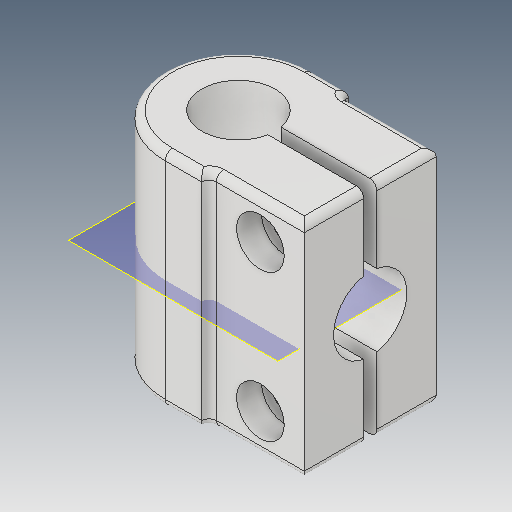
# Autodesk Inventor part: UpperArm_Yawn_Fixture
Saved by Autodesk Inventor 2021.4 (Build 254397000, 397)
## iProperties
Created: 2022-07-06
Part Number: UpperArm_Yawn_Fixture
Material: PBT Plastic
Document SubType Name: Modeling
Designer: alexw
Density: 1.31 g/cm^3
Appearance: Smooth - White
Mass: 13.7456 g
Surface Area: 52.7567 cm^2
Volume: 10.4928 cm^3
Author: alexw
Autodesk Inventor part; units mm, degrees
note: some values were not read from the file. Chosen so that the rebuilt part matches the saved one: direction of "Hole2".
ref_plane "YZ Plane" through (0, 0, 0) normal (1, 0, 0) x (0, 1, 0)
ref_plane "XZ Plane" through (0, 0, 0) normal (0, 1, 0) x (-1, 0, 0)
ref_plane "XY Plane" through (0, 0, 0) normal (0, 0, 1) x (1, 0, 0)
sketch "Sketch1" plane through (0, 0, 0) normal (0, 0, 1) x (1, 0, 0)
  line L0 (28, 30.2) -> (0, 30.2)
  line L1 (0, 30.2) -> (0, 0)
  line L2 (0, 15.1) -> (28, 15.1) construction
  line L3 (28, 0) -> (28, 30.2)
  line L4 (0, 0) -> (28, 0)
  line L5 (20, 15.1) -> (20, 30.2) construction
  dimension "d0" = 30.2
  dimension "d3" = 28
  dimension "d26" = 20
  dimension "d27" = 8
  constraints: 12 end point, 2 midpoint, 2 parallel, 2 perpendicular, 2 point on line, 1 horizontal, 1 symmetric about line
  measures "d0" distance of L0.end L1.end
  measures "d3" distance between parallel lines of L3 L1
  measures "d26" distance between parallel lines of L1 L5
  measures "d27" distance between parallel lines of L3 L5
extrude "Extrusion1" add sketch "Sketch1" along normal blind 20
sketch "Sketch2" plane through (0, 30.2, 0) normal (0, 1, 0) x (1, 0, 0)
  line L0 (0, 0) -> (0, -20) construction
  line L1 (0, 0) -> (28, 0) construction
  line L2 (10, -10) -> (0, -10) construction
  line L3 (0, 0) -> (0, -20) construction
  dimension "d48" = 10
  constraints: 2 end point, 1 horizontal, 1 midpoint
  measures "d48" distance from line of L0 L2.start
hole "Hole1" at (10, 30.2, 10) direction (0, -1, 0) diameter 10 end through all
sketch "Sketch3" plane through (0, 0, 0) normal (0, -1, 0) x (1, 0, 0)
  line L0 (28, 20) -> (15, 20)
  line L1 (16, 19) -> (28, 19)
  line L2 (28, 19) -> (28, 20)
  circle A0 centre (16, 20) radius 1 construction
  arc A1 (15, 20) -> (16, 19) centre (16, 20) ccw
  circle A2 centre (10, 10) radius 5 construction
  line L3 (15, 10) -> (15, 20) construction
  line L4 (0, 20) -> (28, 20) construction
  line L5 (28, 0) -> (28, 20) construction
  line L6 (10, 10) -> (15, 10) construction
  line L7 (28, 0) -> (15, 0)
  line L8 (16, 1) -> (28, 1)
  line L9 (28, 1) -> (28, 0)
  arc A3 (16, 1) -> (15, 0) centre (16, 0) ccw
  point P0 (0, 0)
  dimension "d15" = 2
  dimension "d46" = 18
  constraints: 16 end point, 7 symmetric about line, 6 point on circle, 3 centre point, 2 collinear, 2 concentric, 2 horizontal, 2 tangent, 1 horizontal alignment, 1 parallel, 1 perpendicular, 2 other
  measures "d15" diameter of A0
  measures "d46" diameter of L1 L6
extrude "Extrusion2" cut sketch "Sketch3" against normal through all
fillet "Fillet1" radius 10 2 edges at (0, 15.1, 0) (0, 15.1, 20)
sketch "Sketch4" plane through (15, 30.2, 20) normal (0, 1, 0) x (1, 0, 0)
  circle A0 centre (-5, 10) radius 5 construction
  line L0 (-5, 10) -> (13, 10) construction
  line L1 (-5, 10.9) -> (13, 10.9)
  line L2 (13, 10.9) -> (13, 9.1)
  line L3 (13, 9.1) -> (-5, 9.1)
  line L4 (-5, 9.1) -> (-5, 10.9)
  line L5 (-5, 10.9) -> (13, 9.1) construction
  line L6 (13, 10.9) -> (-5, 9.1) construction
  line L7 (13, 19) -> (13, 1) construction
  point P0 (4, 10)
  point P1 (12, 15)
  point P2 (13, 1)
  point P3 (12, 18)
  dimension "d19" = 1.8
  constraints: 14 end point, 3 midpoint, 2 horizontal, 2 parallel, 1 perpendicular, 1 vertical, 2 other
  measures "d19" distance of L3.end L1.start
extrude "Extrusion3" cut sketch "Sketch4" against normal through all
sketch "Sketch5" plane through (28, 0, 19) normal (1, 0, 0) x (0, 0, -1)
  circle A0 centre (9, 15.1) radius 5
  line L0 (0, 0) -> (0, 30.2) construction
  line L1 (0, 0) -> (18, 30.2) construction
  line L2 (18, 0) -> (0, 30.2) construction
  line L3 (18, 0) -> (18, 30.2) construction
  dimension "d22" = 10
  constraints: 4 end point, 1 centre point, 1 coincident, 1 midpoint
  measures "d22" diameter of A0
extrude "Extrusion4" cut sketch "Sketch5" against normal up to surface
sketch "Sketch6" plane through (16, 0, 19) normal (0, 0, 1) x (1, 0, 0)
  line L0 (0, 30.2) -> (12, 30.2) construction
  line L1 (0, 0) -> (0, 30.2) construction
  line L2 (12, 0) -> (0, 0) construction
  line L3 (12, 30.2) -> (12, 0) construction
  line L4 (6, 0) -> (6, 30.2) construction
  line L5 (6, 15.1) -> (0, 15.1) construction
  point P0 (-16, 0)
  point P1 (6, 5.1)
  point P2 (6, 25.1)
  dimension "d28" = 10
  constraints: 4 end point, 4 midpoint, 1 horizontal, 1 point on line, 1 symmetric about line, 1 vertical
  measures "d28" distance from line of point (6, 5.1) L5
hole "Hole2" at (22, 5.1, 19) at (22, 25.1, 19) direction (0, 0, -1) diameter 3.4 depth 8.1 counterbore diameter 6.5 counterbore depth 3.4 clearance for "Socket Head Cap Screw ISO 4762" size "M3" standard "ISO"
sketch "Sketch7" plane through (14.9183, 30.2, 9.1) normal (0, 0, 1) x (1, 0, 0)
  point P0 (-14.9183, -30.2)
  point P1 (7.0817, -5.1)
  point P2 (7.0817, -25.1)
hole "Hole3" at (22, 25.1, 9.1) at (22, 5.1, 9.1) direction (0, 0, -1) diameter 2.459 depth 8.8 tip angle 118 thread size "M3x0.5" class "6H" standard "ISO Metric profile"
ref_plane "Work Plane1" through (16, 15.1, 19) normal (0, -1, 0) x (1, 0, 0)
fillet "Fillet2" radius 1 18 edges at (15.2929, 30.2, 19.2929) (22, 30.2, 19) (2.9289, 30.2, 2.9289) (12.4999, 30.2, 0) (12.4999, 30.2, 20) (15.2929, 30.2, 0.7071) (22, 30.2, 1) (15.2929, 0, 19.2929) (22, 0, 19) (12.4999, 0, 20) (12.4999, 0, 0) (2.9289, 0, 2.9289) (15.2929, 0, 0.7071) (22, 0, 1) (28, 0, 5.05) (28, 0, 14.95) (28, 30.2, 14.95) (28, 30.2, 5.05)
equation "\"d0\" = YawnFixation_Width"
equation "\"d26\" = YawnShaft_Diameter + Aufmass_ShaftFixationSide"
equation "\"d4\" = YawnShaft_Diameter + Aufmass_ShaftFixationSide"
equation "\"d48\" = 0.5 * d4"
equation "\"d7\" = YawnShaft_Diameter"
equation "\"d18\" = 0.5 * d4"
equation "\"d22\" = Shaft_DiaOut"
equation "\"Aufmass_ShaftFixationSide\" = 10"
equation "\"YawnFixation_Width\" = 30.2"
equation "\"YawnShaft_Diameter\" = 10"
equation "\"Shaft_DiaOut\" = 10"
body "Solid1"
